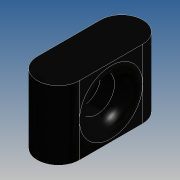
# Autodesk Inventor part: P101Bielle
Saved by Autodesk Inventor 2015 SP1 (Build 190203100, 203)
## iProperties
Created: 2016-10-17
Part Number: P101Bielle
Material: ABS Plastic
Document SubType Name: Modeling
Designer: serge.amoos
Density: 1.06 g/cm^3
Appearance: Smooth - Black
Author: serge.amoos
Autodesk Inventor part; units mm, degrees
ref_plane "YZ Plane" through (0, 0, 0) normal (1, 0, 0) x (0, 1, 0)
ref_plane "XZ Plane" through (0, 0, 0) normal (0, 1, 0) x (-1, 0, 0)
ref_plane "XY Plane" through (0, 0, 0) normal (0, 0, 1) x (1, 0, 0)
sketch "Sketch1" plane through (0, 0, 0) normal (0, 0, 1) x (1, 0, 0)
  line L0 (-4.2, 0) -> (4.2, 0) projected
  line L1 (0, -1.5) -> (0, 9) projected
  line L2 (-3, 7.5) -> (3, 7.5)
  line L3 (3, 7.5) -> (3, 0)
  line L4 (3, 0) -> (-3, 0)
  line L5 (-3, 0) -> (-3, 7.5)
  point P0 (0, 0)
  point P1 (0, 0)
  dimension "d0" = 6
  dimension "d1" = 7.5
  constraints: 8 end point, 2 parallel, 2 point on line, 1 horizontal, 1 midpoint, 1 perpendicular
  measures "d0" distance of L2.start L2.end
  measures "d1" distance between parallel lines of L0 L2
extrude "Extrusion1" add sketch "Sketch1" along normal mid plane 9.8
fillet "Fillet1" radius 3 2 edges at (3, 7.5, 0) (-3, 7.5, 0)
mirror "Mirror1" about plane through (-3, 0, 0) normal (0, -1, 0)
sketch "Sketch2" plane through (3, 4.5, 4.9) normal (1, 0, 0) x (0, 0, -1)
  point P0 (4.9, -4.5)
hole "Hole1" at (3, 0, 0) direction (-1, 0, 0) diameter 5 end through all
fillet "Fillet2" radius 2 2 edges at (3, 0, 2.5) (-3, 0, 2.5)
body "Solid1"
